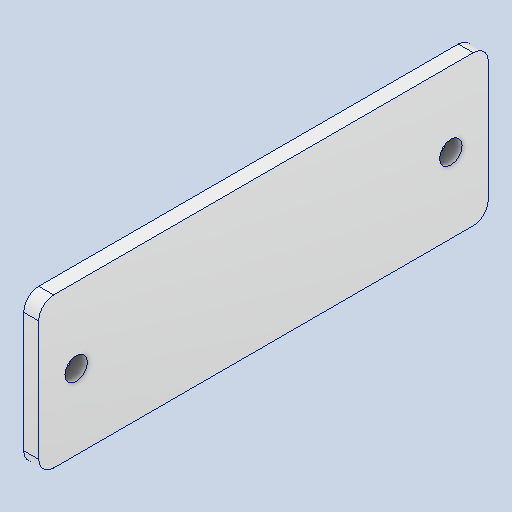
# Autodesk Inventor part: base_weel-v1-Plate-expand-1
Saved by Autodesk Inventor 2025.1 (Build 291241000, 241)
## iProperties
Created: 2024-12-09
Part Number: base_weel-v1-Plate-expand-1
Material: アルミニウム 6061
Document SubType Name: Modeling
Designer: haruy
Density: 2.7 g/cm^3
Appearance: アルミニウム - フラット
Author: haruy
Autodesk Inventor part; units mm, degrees
ref_plane "YZ Plane" through (0, 0, 0) normal (1, 0, 0) x (0, 1, 0)
ref_plane "XZ Plane" through (0, 0, 0) normal (0, 1, 0) x (-1, 0, 0)
ref_plane "XY Plane" through (0, 0, 0) normal (0, 0, 1) x (1, 0, 0)
sketch "スケッチ1" plane through (0, 0, 0) normal (1, 0, 0) x (0, 1, 0)
  line L0 (-78.1013, 9.4232) -> (-98.1013, 9.4232)
  line L1 (-98.1013, 9.4232) -> (-78.1013, 9.4232)
  line L2 (-78.1013, 9.4232) -> (-78.1013, -630.5768)
  line L3 (-78.1013, -630.5768) -> (-98.1013, -630.5768)
  line L4 (-98.1013, -630.5768) -> (-98.1013, 9.4232)
  line L5 (90.8987, -620.5768) -> (110.8987, -620.5768)
  line L6 (110.8987, -620.5768) -> (110.8987, -53.5768)
  line L7 (110.8987, -53.5768) -> (90.8987, -53.5768)
  line L8 (90.8987, -53.5768) -> (90.8987, -620.5768)
  line L9 (90.8987, 19.4232) -> (90.8987, 586.4232)
  line L10 (-73.5639, 640.5027) -> (90.8987, -49.1588)
  line L11 (90.8987, -49.1588) -> (110.3532, -44.5196)
  line L12 (110.3532, -44.5196) -> (-54.1094, 645.142)
  line L13 (-54.1094, 645.142) -> (-73.5639, 640.5027)
  line L14 (-78.1013, 644.9232) -> (-78.1013, 9.4232)
  circle A0 centre (-88.1013, 639.9232) radius 1.5
  circle A1 centre (-88.1013, 639.9232) radius 1.5
  circle A2 centre (-88.1013, 629.9232) radius 1.5
  circle A3 centre (-88.1013, 629.9232) radius 1.5
  line L15 (-98.1013, 9.4232) -> (-98.1013, 644.9232)
  line L16 (-98.1013, 624.9232) -> (-78.1013, 624.9232)
  line L17 (-78.1013, 624.9232) -> (-67.7648, 616.1846)
  line L18 (-67.7648, 616.1846) -> (-48.3103, 620.8239)
  line L19 (-78.1013, 644.9232) -> (-54.1094, 645.142)
  circle A4 centre (-61.517, 633.0951) radius 1.5
  circle A5 centre (-59.1973, 623.3679) radius 1.5
  line L20 (-78.1013, 644.9232) -> (-98.1013, 644.9232)
  line L21 (-78.1013, 644.9232) -> (-98.1013, 644.9232)
  line L22 (-98.1013, 644.9232) -> (-98.1013, 624.9232)
  line L23 (-98.1013, -20.5768) -> (-78.1013, -20.5768)
  circle A6 centre (-88.1013, -15.5768) radius 1.5
  line L24 (-98.1013, 39.4232) -> (-78.1013, 39.4232)
  circle A7 centre (-88.1013, 34.4232) radius 1.5
  line L25 (-98.1013, 39.4232) -> (-98.1013, 8.2286)
  line L26 (-78.1013, 39.4232) -> (-78.1013, 9.4232)
  point P0 (0, 0)
  point P1 (-78.1013, 19.4232)
  point P2 (-88.1013, -605.5768)
  point P3 (100.8987, -605.5768)
  point P4 (100.8987, -58.5768)
  point P5 (100.8987, -68.5768)
  point P6 (100.8987, -620.5768)
  point P7 (98.3063, -37.112)
  point P8 (95.9867, -27.3847)
  point P9 (-58.0375, 618.5042)
  dimension "d0" = 20
  dimension "d1" = 640
  dimension "d2" = 20
  dimension "d3" = 567
  dimension "d4" = 10
  dimension "d5" = 0
  dimension "d6" = 25
  dimension "d7" = 15
  dimension "d8" = 10
  dimension "d9" = 10
  dimension "d10" = 5
  dimension "d11" = 10
  dimension "d12" = 10
  dimension "d13" = 10
  dimension "d14" = 20
  dimension "d15" = 709
  dimension "d16" = 4.4179
  dimension "d17" = 4.5374
  dimension "d18" = 10
  dimension "d19" = 10
  dimension "d20" = 10
  dimension "d21" = 10
  dimension "d22" = 10
  dimension "d23" = 10
  dimension "d24" = 10
  dimension "d25" = 10
  dimension "d26" = 25
  dimension "d27" = 10
  dimension "d28" = 3
  dimension "d29" = 3
  dimension "d30" = 5
  dimension "d31" = 5
  dimension "d32" = 3
  dimension "d33" = 3
  dimension "d34" = 5
  dimension "d35" = 3
  dimension "d36" = 5
  constraints: 54 end point, 10 point on line, 8 centre point, 8 perpendicular, 7 equal length, 5 coincident, 2 horizontal, 2 midpoint
  measures "d0" distance of L2.end L3.end
  measures "d1" distance between parallel lines of L3 L0
  measures "d2" distance of L7.end L6.end
  measures "d3" distance of L6.end L5.end
  measures "d4" distance between parallel lines of L3 L5
  measures "d5" distance between parallel lines of L9 L8
  measures "d6" distance from line of point (-88.101, -605.577) L3
  measures "d7" distance of point (100.899, -605.577) point (100.899, -620.577)
  measures "d8" distance from line of point (100.899, -605.577) L8
  measures "d9" distance from line of point (-88.101, -605.577) L4
  measures "d10" distance from line of point (100.899, -58.577) L7
  measures "d11" distance of point (100.899, -58.577) point (100.899, -68.577)
  measures "d12" distance from line of point (100.899, -58.577) L8
  measures "d13" distance from line of L8 point (100.899, -68.577)
  measures "d14" distance of L11.end L10.end
  measures "d15" distance of L11.end L12.end
  measures "d16" distance from line of L7 L10.end
  measures "d17" distance from line of L14 L10.start
  measures "d18" distance from line of point (98.306, -37.112) L11
  measures "d19" distance of point (95.987, -27.385) point (98.306, -37.112)
  measures "d20" distance from line of point (95.987, -27.385) L10
  measures "d21" distance from line of point (98.306, -37.112) L10
  measures "d22" distance from line of L10 point (-61.517, 633.095)
  measures "d23" distance from line of L13 point (-61.517, 633.095)
  measures "d24" distance of point (-61.517, 633.095) point (-59.197, 623.368)
  measures "d25" distance from line of L10 point (-59.197, 623.368)
  measures "d26" distance from line of point (-88.101, -15.577) L0
  measures "d27" distance from line of point (-88.101, -15.577) L4
  measures "d28" diameter of A1
  measures "d29" diameter of A3
  measures "d30" distance from line of L16 A2.centre
  measures "d31" distance of point (-58.038, 618.504) point (-59.197, 623.368)
  measures "d32" diameter of A4
  measures "d33" diameter of A5
  measures "d34" distance from line of L23 point (-88.101, -15.577)
  measures "d35" diameter of A6
  measures "d36" distance from line of A7.centre L24
extrude "押し出し1" add sketch "スケッチ1" against normal blind 2 contours L2 L23 L4 L0 | L0 L15 L24 L14
fillet "フィレット1" radius 2 4 edges at (-1, -78.1013, 39.4232) (-1, -98.1013, 39.4232) (-1, -98.1013, -20.5768) (-1, -78.1013, -20.5768)
equation "\"d21\" = d20"
